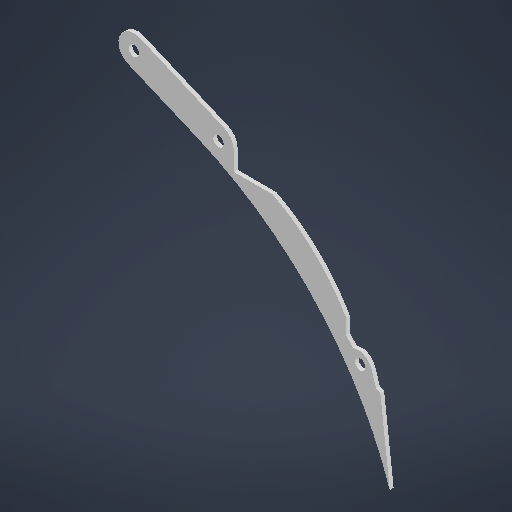
# Autodesk Inventor part: ramp
Saved by Autodesk Inventor 2025.2 (Build 292293000, 293)
## iProperties
Created: 2025-01-15
Part Number: ramp
Material: Generic
Document SubType Name: Modeling
Designer: Jahan
Density: 1 g/cm^3
Appearance: Default
Author: Jahan
Autodesk Inventor part; units mm, degrees
ref_plane "YZ Plane" through (0, 0, 0) normal (1, 0, 0) x (0, 1, 0)
ref_plane "XZ Plane" through (0, 0, 0) normal (0, 1, 0) x (-1, 0, 0)
ref_plane "XY Plane" through (0, 0, 0) normal (0, 0, 1) x (1, 0, 0)
sketch "Sketch1" plane through (0, 0, 0) normal (0, 0, 1) x (1, 0, 0)
  circle A0 centre (41.9247, 14.1753) radius 2.1844
  ellipse E0 centre (-16.8128, 64.9442) end of major axis (-18.9972, 64.9442) minor radius 2.1844
  ellipse E1 centre (-51.9254, 79.8172) end of major axis (-49.741, 79.8172) minor radius 2.1844
  line L0 (-19.2895, 59.0971) -> (-54.4021, 73.9701)
  line L1 (-49.4488, 85.6642) -> (-14.3361, 70.7913)
  line L2 (-10.4628, 64.9442) -> (-10.4628, 57.0349)
  line L3 (48.47, 8.8519) -> (46.6593, 14.6816)
  line L4 (50.2722, 8.0885) -> (48.47, 8.8519)
  line L5 (38.9963, 18.7191) -> (36.0653, 21.6265)
  line L6 (38.9963, 18.7191) -> (41.9273, 18.9148)
  line L7 (36.0653, 21.6265) -> (36.0653, 27.9765)
  arc A1 (36.0653, 27.9765) -> (5.6382, 57.0349) centre (-28.0473, -8.6966) ccw
  line L8 (5.6382, 57.0349) -> (-10.4628, 57.0349)
  arc A2 (-49.4488, 85.6642) -> (-54.4021, 73.9701) centre (-51.9254, 79.8172) ccw
  arc A3 (-10.4628, 64.9442) -> (-14.3361, 70.7913) centre (-16.8128, 64.9442) ccw
  arc A4 (46.6593, 14.6816) -> (41.9273, 18.9148) centre (40.7609, 12.8496) ccw
  arc A5 (54.1461, -24.7627) -> (54.1954, -24.7517) centre (54.1702, -24.7547) ccw
  arc A6 (54.1431, -24.7536) -> (-25.7804, 61.8465) centre (-81.5487, -69.803) ccw
  line L9 (54.1461, -24.7627) -> (54.1431, -24.7536)
  line L10 (54.1954, -24.7517) -> (50.2722, 8.0885)
  point P0 (0, 0)
  point P1 (54.2254, -25.0022)
  point P2 (54.1431, -24.7536)
  dimension "d3" = 6.35
  dimension "d4" = 0.0254
  constraints: 22 end point, 12 point on circle, 8 centre point, 2 coincident, 2 vertical, 1 horizontal, 1 point on line, 1 tangent, 3 other
  measures "d3" distance of L7.start L7.end
  measures "d4" radius of A5
extrude "Extrusion1" add sketch "Sketch1" along normal blind 1.5875
body "Solid1"
